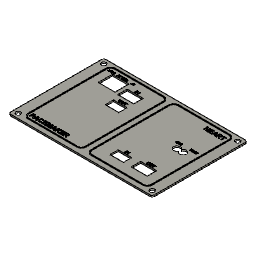
testing_station_casing_top v22 (Autodesk Fusion 360 design; units mm, degrees)
Autodesk Fusion 360 part; units mm, degrees
(part 1 of 2)
sketch "Sketch1" plane through (0, 0, 0) normal (0, 0, 1) x (1, 0, 0)
  line L0 (0, 0) -> (148, 0)
  line L1 (148, 0) -> (148, 98)
  line L2 (148, 98) -> (0, 98)
  line L3 (0, 98) -> (0, 0)
  dimension "d1" = 148
  dimension "d2" = 98
  constraint horizontal L0
  constraint vertical L1
  constraint horizontal L2
  constraint vertical L3
  constraint coincident L0.start L3.end
  measures "d1" distance of L0.start L0.end
  measures "d2" distance of L0.start L2.end
extrude "Extrude1" add sketch "Sketch1" along normal blind 1.5
sketch "Sketch2" plane through (0, 0, 1.5) normal (0, 0, 1) x (-1, 0, 0)
  line L0 (0, -98) -> (0, 0)
  line L1 (0, 0) -> (-148, 0)
  line L2 (-148, 0) -> (-148, -98)
  line L3 (-148, -98) -> (0, -98)
  line L4 (-7.1651, -89.25) -> (-2.8349, -89.25)
  line L5 (0, 0) -> (-148, 0)
  line L6 (-2.8349, -96.75) -> (-7.1651, -96.75)
  line L7 (0, -98) -> (0, 0)
  line L8 (-148, -98) -> (0, -98)
  line L9 (-2.8349, -89.25) -> (-0.6699, -93)
  line L10 (-9.3301, -93) -> (-7.1651, -89.25)
  line L11 (-148, 0) -> (-148, -98)
  line L12 (-0.6699, -93) -> (-2.8349, -96.75)
  line L13 (-7.1651, -96.75) -> (-9.3301, -93)
  circle A0 centre (-5, -93) radius 2.45
  circle A1 centre (-5, -5) radius 2.45
  circle A2 centre (-143, -5) radius 2.45
  circle A3 centre (-143, -93) radius 2.45
  dimension "d5" = 4.9
  dimension "d10" = 7.5
  dimension "d11" = 7.5
  dimension "d12" = 120
  dimension "d13" = 120
  dimension "d26" = 5
  dimension "d27" = 5
  dimension "d34" = 4.9
  dimension "d35" = 4.9
  dimension "d36" = 4.9
  dimension "d37" = 5
  dimension "d38" = 5
  dimension "d39" = 5
  dimension "d40" = 5
  dimension "d41" = 5
  dimension "d42" = 5
  dimension "d97" = 3.75
  dimension "d98" = 3.75
  dimension "d99" = 3.75
  constraint horizontal L6
  constraint parallel L4 L6
  constraint parallel L10 L12
  constraint parallel L9 L13
  constraint coincident L2.end L3.start
  constraint coincident L1.end L2.start
  constraint coincident L0.start L3.end
  constraint coincident L0.end L1.start
  constraint equal L9 L13
  measures "d5" diameter of A0
  measures "d10" distance of L10 L12
  measures "d11" distance of L9 L13
  measures "d12" angle of L4 L10
  measures "d13" angle of L6 L13
  measures "d26" distance of A0.centre L7
  measures "d27" distance of A0.centre L8
  measures "d34" diameter of A3
  measures "d35" diameter of A1
  measures "d36" diameter of A2
  measures "d37" distance of L11 A3.centre
  measures "d38" distance of L8 A3.centre
  measures "d39" distance of L11 A2.centre
  measures "d40" distance of L5 A2.centre
  measures "d41" distance of L5 A1.centre
  measures "d42" distance of L7 A1.centre
  measures "d97" distance of A0.centre L6
  measures "d98" distance of A0.centre L12
  measures "d99" distance of A0.centre L9
extrude "Extrude2" cut sketch "Sketch2" along normal through all and the other way through all contours A0 | A1 | A2 | A3
sketch "Sketch3" plane through (0, 0, 1.5) normal (0, 0, 1) x (-1, 0, 0)
  circle A0 centre (-5, -5) radius 2.45
  circle A1 centre (-5, -93) radius 2.45
  line L0 (0, -98) -> (0, 0)
  line L1 (-22.5, -92.78) -> (-22.5, -86.78)
  line L2 (-15, -86.78) -> (-15, -92.78)
  line L3 (-44.6822, -95.28) -> (-44.6822, -73.28)
  line L4 (-28.9322, -95.28) -> (-44.6822, -95.28)
  line L5 (-55.9389, -86.78) -> (-48.4389, -86.78)
  line L6 (-48.4389, -86.78) -> (-48.4389, -92.78)
  circle A2 centre (-12.8194, -22.6238) radius 1.5
  line L7 (-44.6822, -73.28) -> (-28.9322, -73.28)
  line L8 (-28.9322, -73.28) -> (-28.9322, -95.28)
  line L9 (-15, -92.78) -> (-22.5, -92.78)
  circle A3 centre (-59.7586, -77.5513) radius 1.5
  line L10 (-48.4389, -92.78) -> (-55.9389, -92.78)
  line L11 (-22.5, -86.78) -> (-15, -86.78)
  line L12 (-63.34, -10) -> (-10, -10)
  line L13 (-63.34, -91.28) -> (-63.34, -10)
  circle A4 centre (-12.8194, -76.3321) radius 1.5
  line L14 (-55.9389, -92.78) -> (-55.9389, -86.78)
  circle A5 centre (-59.7586, -22.6238) radius 1.5
  line L15 (-10, -91.28) -> (-63.34, -91.28)
  line L16 (-10, -10) -> (-10, -91.28)
  line L17 (0, 0) -> (-148, 0)
  line L18 (-148, 0) -> (-148, -98)
  line L19 (-148, -98) -> (0, -98)
  line L20 (0, -98) -> (0, 0)
  line L21 (-70.214, -90.398) -> (-140, -90.398)
  line L22 (-140, -90.398) -> (-140, -10)
  line L23 (-70.214, -10) -> (-70.214, -90.398)
  line L24 (-114.82, -91.7786) -> (-124.1322, -91.7786)
  line L25 (-124.1322, -91.7786) -> (-124.1322, -84.0185)
  line L26 (-124.1322, -84.0185) -> (-114.82, -84.0185)
  line L27 (-114.82, -84.0185) -> (-114.82, -91.7786)
  line L28 (-81.756, -10) -> (-83.5436, -8)
  line L29 (-83.5436, -8) -> (-116.4586, -8)
  line L30 (-116.4586, -8) -> (-118.458, -10)
  line L31 (-140, -10) -> (-118.458, -10)
  line L32 (-81.756, -10) -> (-70.214, -10)
  circle A6 centre (-113.89, -10.5) radius 1.5
  circle A7 centre (-129.13, -61.198) radius 1.5
  circle A8 centre (-81.084, -62.468) radius 1.5
  circle A9 centre (-129.13, -57.642) radius 1
  line L33 (-133.506, -56.3529) -> (-136.9699, -56.3529) construction
  line L34 (-136.9699, -56.3529) -> (-136.9699, -58.3529) construction
  line L35 (-136.9699, -58.3529) -> (-133.506, -58.3529) construction
  line L36 (-133.506, -58.3529) -> (-133.506, -56.3529) construction
  circle A10 centre (-60.6896, -73.1803) radius 1
  line L37 (-55.7149, -72.2742) -> (-59.1788, -72.2742) construction
  line L38 (-59.1788, -72.2742) -> (-59.1788, -74.2742) construction
  line L39 (-59.1788, -74.2742) -> (-55.7149, -74.2742) construction
  line L40 (-55.7149, -74.2742) -> (-55.7149, -72.2742) construction
  point P0 (-148, -98)
  dimension "d45" = 3
  dimension "d46" = 3
  dimension "d60" = 4
  dimension "d61" = 15.75
  dimension "d62" = 7.4011
  dimension "d63" = 53.34
  dimension "d64" = 81.28
  dimension "d65" = 18.6578
  dimension "d68" = 2.8194
  dimension "d69" = 14.9479
  dimension "d70" = 12.6238
  dimension "d73" = 2.8194
  dimension "d74" = 6
  dimension "d75" = 22
  dimension "d76" = 7.5
  dimension "d78" = 5
  dimension "d155" = 10
  dimension "d156" = 10
  dimension "d157" = 3
  dimension "d158" = 3
  dimension "d159" = 3.5814
  dimension "d160" = 54.9275
  dimension "d161" = 12.6238
  dimension "d162" = 3.5814
  dimension "d163" = 7.5
  dimension "d164" = 1.5
  dimension "d165" = 6
  dimension "d166" = 69.786
  dimension "d167" = 8
  dimension "d168" = 80.398
  dimension "d169" = 2
  dimension "d170" = 21.542
  dimension "d171" = 32.915
  dimension "d172" = 11.542
  dimension "d173" = 2.828
  dimension "d174" = 10.87
  dimension "d175" = 10.87
  dimension "d176" = 27.93
  dimension "d177" = 29.2
  dimension "d178" = 3
  dimension "d179" = 3
  dimension "d180" = 3
  dimension "d181" = 2.5
  dimension "d182" = 26.11
  dimension "d183" = 10
  dimension "d184" = 2
  dimension "d186" = 3.556
  dimension "d204" = 2
  dimension "d206" = 0.931
  dimension "d207" = 4.371
  constraint horizontal L15
  constraint vertical L13
  constraint horizontal L12
  constraint vertical L16
  constraint horizontal L10
  constraint vertical L14
  constraint horizontal L5
  constraint vertical L6
  constraint horizontal L4
  constraint vertical L3
  constraint horizontal L7
  constraint vertical L8
  constraint horizontal L9
  constraint horizontal L11
  constraint vertical L2
  constraint collinear L9 L10
  constraint collinear L5 L11
  constraint coincident L0.end L17.start
  constraint horizontal L17
  constraint vertical L18
  constraint horizontal L19
  constraint vertical L20
  constraint coincident P0 L18.end
  constraint horizontal L21
  constraint vertical L22
  constraint horizontal L31
  constraint vertical L23
  constraint horizontal L24
  constraint vertical L25
  constraint horizontal L26
  constraint vertical L27
  constraint coincident L28.start L31
  constraint collinear L31 L32
  constraint perpendicular L33 L34
  constraint parallel L33 L35
  constraint parallel L34 L36
  constraint vertical A7.centre A9.centre
  constraint perpendicular L37 L38
  constraint parallel L37 L39
  constraint parallel L38 L40
  measures "d45" diameter of A4
  measures "d46" diameter of A2
  measures "d60" distance of L4 L15
  measures "d61" distance of L4.start L3.start
  measures "d62" distance of L13 L14
  measures "d63" distance of L13.start L15.start
  measures "d64" distance of L15.start L12.end
  measures "d65" distance of L3 L13
  measures "d68" distance of A4.centre L16
  measures "d69" distance of A4.centre L15
  measures "d70" distance of A2.centre L12
  measures "d73" distance of A2.centre L16
  measures "d74" distance of L10.end L5.start
  measures "d75" distance of L7.end L4.start
  measures "d76" distance of L10.end L6.end
  measures "d78" distance of L2 L16
  measures "d155" distance of L16 L20
  measures "d156" distance of L12 L17
  measures "d157" diameter of A5
  measures "d158" diameter of A3
  measures "d159" distance of A3.centre L13
  measures "d160" distance of A3.centre A5.centre
  measures "d161" distance of A5.centre L12
  measures "d162" distance of A5.centre L13
  measures "d163" distance of L1.start L2.end
  measures "d164" distance of L9 L15
  measures "d165" distance of L1.end L1.start
  measures "d166" distance of L21.start L21.end
  measures "d167" distance of L18 L22
  measures "d168" distance of L21.end L22.end
  measures "d169" distance of L29 L31
  measures "d170" distance of L22 L30.end
  measures "d171" distance of L28.end L29.end
  measures "d172" distance of L23 L28.start
  measures "d173" distance of L29.end L30.end
  measures "d174" distance of L22 A7.centre
  measures "d175" distance of L23 A8.centre
  measures "d176" distance of L21 A8.centre
  measures "d177" distance of L21 A7.centre
  measures "d178" diameter of A8
  measures "d179" diameter of A7
  measures "d180" diameter of A6
  measures "d181" distance of L29 A6.centre
  measures "d182" distance of L22 A6.centre
  measures "d183" distance of L17 L31
  measures "d184" diameter of A9
  measures "d186" distance of A7.centre A9.centre
  measures "d204" diameter of A10
  measures "d206" horizontal distance of A3.centre A10.centre
  measures "d207" vertical distance of A3.centre A10.centre
sketch "Sketch4" plane through (0, 0, 1.5) normal (0, 0, 1) x (-1, 0, 0)
  line L0 (-41.7296, -80.5083) -> (-54.1296, -80.5083)
  line L1 (-54.1296, -80.5083) -> (-54.1296, -74.7583)
  line L2 (-54.1296, -74.7583) -> (-41.7296, -74.7583)
  line L3 (-41.7296, -74.7583) -> (-41.7296, -80.5083)
  line L4 (-44.2616, -63.8513) -> (-54.1616, -63.8513)
  line L5 (-54.1616, -63.8513) -> (-54.1616, -59.3513)
  line L6 (-54.1616, -59.3513) -> (-44.2616, -59.3513)
  line L7 (-44.2616, -59.3513) -> (-44.2616, -63.8513)
  line L8 (-113.193, -22.958) -> (-125.593, -22.958)
  line L9 (-125.593, -22.958) -> (-125.593, -17.208)
  line L10 (-125.593, -17.208) -> (-113.193, -17.208)
  line L11 (-113.193, -17.208) -> (-113.193, -22.958)
  line L12 (-91.149, -21.75) -> (-101.049, -21.75)
  line L13 (-101.049, -21.75) -> (-101.049, -17.25)
  line L14 (-101.049, -17.25) -> (-91.149, -17.25)
  line L15 (-91.149, -17.25) -> (-91.149, -21.75)
  line L16 (-103.049, -23.75) -> (-103.049, -15.25)
  line L17 (-103.049, -15.25) -> (-89.149, -15.25)
  line L18 (-89.149, -15.25) -> (-89.149, -23.75)
  line L19 (-89.149, -23.75) -> (-103.049, -23.75)
  line L20 (-111.193, -15.208) -> (-111.193, -24.958)
  line L21 (-111.193, -24.958) -> (-127.593, -24.958)
  line L22 (-127.593, -24.958) -> (-127.593, -15.208)
  line L23 (-127.593, -15.208) -> (-111.193, -15.208)
  line L24 (-39.7296, -72.7583) -> (-39.7296, -82.5083)
  line L25 (-39.7296, -82.5083) -> (-56.1296, -82.5083)
  line L26 (-56.1296, -82.5083) -> (-56.1296, -72.7583)
  line L27 (-56.1296, -72.7583) -> (-39.7296, -72.7583)
  line L28 (-42.2616, -65.8513) -> (-56.1616, -65.8513)
  line L29 (-56.1616, -65.8513) -> (-56.1616, -57.3513)
  line L30 (-56.1616, -57.3513) -> (-42.2616, -57.3513)
  line L31 (-42.2616, -57.3513) -> (-42.2616, -65.8513)
  line L32 (-20.8196, -75.5813) -> (-34.0196, -75.5813)
  line L33 (-34.0196, -75.5813) -> (-34.0196, -86.0963)
  line L34 (-34.0196, -86.0963) -> (-20.8196, -86.0963)
  line L35 (-20.8196, -86.0963) -> (-20.8196, -75.5813)
  line L36 (-36.0196, -88.0963) -> (-18.8196, -88.0963)
  line L37 (-18.8196, -88.0963) -> (-18.8196, -73.5813)
  line L38 (-18.8196, -73.5813) -> (-36.0196, -73.5813)
  line L39 (-36.0196, -73.5813) -> (-36.0196, -88.0963)
  circle A0 centre (-118.398, -55.077) radius 3.5
  circle A1 centre (-124.685, -55.077) radius 3.5
  point P0 (-129.13, -57.642)
  point P1 (-60.6896, -73.1803)
  dimension "d187" = 3.537
  dimension "d188" = 34.684
  dimension "d189" = 12.144
  dimension "d190" = 12.4
  dimension "d191" = 5.75
  dimension "d192" = 9.9
  dimension "d193" = 4.5
  dimension "d198" = -2
  dimension "d199" = -2
  dimension "d208" = 6.56
  dimension "d209" = 5.75
  dimension "d210" = 12.4
  dimension "d211" = 1.578
  dimension "d212" = 9.329
  dimension "d213" = 4.5
  dimension "d214" = 9.9
  dimension "d215" = 6.528
  dimension "d216" = -2
  dimension "d217" = -2
  dimension "d227" = 13.2
  dimension "d228" = 10.515
  dimension "d229" = 2
  dimension "d230" = 26.67
  dimension "d231" = 2.401
  dimension "d235" = 7
  dimension "d236" = 7
  dimension "d244" = 1.208
  dimension "d245" = 2.565
  dimension "d246" = 4.445
  dimension "d247" = 6.287
  constraint horizontal L0
  constraint vertical L1
  constraint horizontal L2
  constraint vertical L3
  constraint horizontal L4
  constraint vertical L5
  constraint horizontal L6
  constraint vertical L7
  constraint horizontal L8
  constraint vertical L9
  constraint horizontal L10
  constraint vertical L11
  constraint horizontal L12
  constraint vertical L13
  constraint horizontal L14
  constraint vertical L15
  constraint horizontal L32
  constraint vertical L33
  constraint horizontal L34
  constraint vertical L35
  constraint horizontal A0.centre A1.centre
  measures "d187" distance of L9 P0
  measures "d188" distance of L8 P0
  measures "d189" distance of L11 L13
  measures "d190" distance of L8.start L8.end
  measures "d191" distance of L8.start L10.end
  measures "d192" distance of L12.start L12.end
  measures "d193" distance of L12.start L14.end
  measures "d208" distance of L1 P1
  measures "d209" distance of L0.end L1.end
  measures "d210" distance of L0.start L0.end
  measures "d211" distance of L2 P1
  measures "d212" distance of L4 P1
  measures "d213" distance of L4.start L6.end
  measures "d214" distance of L5.end L6.end
  measures "d215" distance of L5 P1
  measures "d227" distance of L32.start L32.end
  measures "d228" distance of L32.start L34.end
  measures "d230" distance of P1 L33
  measures "d231" distance of P1 L32
  measures "d235" diameter of A1
  measures "d236" diameter of A0
  measures "d244" distance of L8 L12
  measures "d245" vertical distance of P0 A1.centre
  measures "d246" horizontal distance of P0 A1.centre
  measures "d247" distance of A0.centre A1.centre
extrude "Extrude3" cut sketch "Sketch4" along normal through all and the other way through all contours L0 L1 L2 L3 | L4 L5 L6 L7 | L8 L9 L10 L11 | L12 L13 L14 L15 | L16 L17 L18 L19 | L20 L21 L22 L23 | L24 L25 L26 L27 | L28 L29 L30 L31 | L32 L33 L34 L35 | L36 L37 L38 L39 | A0 A1 | A0 A1 | A0 A1
sketch "Sketch5" plane through (0, 0, 1.5) normal (0, 0, 1) x (-1, 0, 0)
  circle A0 centre (-5, -5) radius 2.45
  circle A1 centre (-143, -5) radius 2.45
  circle A2 centre (-5, -93) radius 2.45
  circle A3 centre (-143, -93) radius 2.45
  line L0 (0, -98) -> (0, 0)
  line L1 (0, 0) -> (-148, 0)
  line L2 (-148, 0) -> (-148, -98)
  line L3 (-148, -98) -> (0, -98)
  line L4 (-46.2265, -83.5083) -> (-49.6327, -83.5083) construction
  line L5 (-49.6327, -83.5083) -> (-49.6327, -87.5083) construction
  line L6 (-49.6327, -87.5083) -> (-46.2265, -87.5083) construction
  line L7 (-46.2265, -87.5083) -> (-46.2265, -83.5083) construction
  line L8 (-45.1178, -66.8513) -> (-53.3053, -66.8513) construction
  line L9 (-53.3053, -66.8513) -> (-53.3053, -70.8513) construction
  line L10 (-53.3053, -70.8513) -> (-45.1178, -70.8513) construction
  line L11 (-45.1178, -70.8513) -> (-45.1178, -66.8513) construction
  line L12 (-115.2993, -25.958) -> (-123.4868, -25.958) construction
  line L13 (-123.4868, -25.958) -> (-123.4868, -29.958) construction
  line L14 (-123.4868, -29.958) -> (-115.2993, -29.958) construction
  line L15 (-115.2993, -29.958) -> (-115.2993, -25.958) construction
  line L16 (-94.3959, -24.75) -> (-97.8021, -24.75) construction
  line L17 (-97.8021, -24.75) -> (-97.8021, -28.75) construction
  line L18 (-97.8021, -28.75) -> (-94.3959, -28.75) construction
  line L19 (-94.3959, -28.75) -> (-94.3959, -24.75) construction
  line L20 (-22.1066, -89.0963) -> (-32.7326, -89.0963) construction
  line L21 (-32.7326, -89.0963) -> (-32.7326, -92.0963) construction
  line L22 (-32.7326, -92.0963) -> (-22.1066, -92.0963) construction
  line L23 (-22.1066, -92.0963) -> (-22.1066, -89.0963) construction
  line L24 (-13.0194, -89.0963) -> (-19.5277, -89.0963) construction
  line L25 (-19.5277, -89.0963) -> (-19.5277, -92.0963) construction
  line L26 (-19.5277, -92.0963) -> (-13.0194, -92.0963) construction
  line L27 (-13.0194, -92.0963) -> (-13.0194, -89.0963) construction
  line L28 (-36.486, -89.0963) -> (-39.8325, -89.0963) construction
  line L29 (-39.8325, -89.0963) -> (-39.8325, -92.0963) construction
  line L30 (-39.8325, -92.0963) -> (-36.486, -92.0963) construction
  line L31 (-36.486, -92.0963) -> (-36.486, -89.0963) construction
  line L32 (-27.4196, -88.0963) -> (-27.4196, -73.5813)
  line L33 (-127.593, -15.208) -> (-111.193, -15.208)
  line L34 (-111.193, -15.208) -> (-111.193, -24.958)
  line L35 (-111.193, -24.958) -> (-127.593, -24.958)
  line L36 (-127.593, -24.958) -> (-127.593, -15.208)
  line L37 (-89.149, -23.75) -> (-103.049, -23.75)
  line L38 (-103.049, -23.75) -> (-103.049, -15.25)
  line L39 (-103.049, -15.25) -> (-89.149, -15.25)
  line L40 (-89.149, -15.25) -> (-89.149, -23.75)
  line L41 (-89.149, -15.25) -> (-89.149, -23.75)
  line L42 (-42.2616, -57.3513) -> (-42.2616, -65.8513)
  line L43 (-42.2616, -65.8513) -> (-56.1616, -65.8513)
  line L44 (-56.1616, -65.8513) -> (-56.1616, -57.3513)
  line L45 (-56.1616, -57.3513) -> (-42.2616, -57.3513)
  line L46 (-56.1296, -72.7583) -> (-39.7296, -72.7583)
  line L47 (-39.7296, -72.7583) -> (-39.7296, -82.5083)
  line L48 (-39.7296, -82.5083) -> (-56.1296, -82.5083)
  line L49 (-56.1296, -82.5083) -> (-56.1296, -72.7583)
  line L50 (-39.7296, -72.7583) -> (-39.7296, -82.5083)
  line L51 (-42.2616, -57.3513) -> (-42.2616, -65.8513)
  line L52 (-36.0196, -73.5813) -> (-18.8196, -73.5813)
  line L53 (-18.8196, -73.5813) -> (-18.8196, -88.0963)
  line L54 (-18.8196, -88.0963) -> (-36.0196, -88.0963)
  line L55 (-36.0196, -88.0963) -> (-36.0196, -73.5813)
  line L56 (-111.398, -60.077) -> (-117.398, -60.077) construction
  line L57 (-117.398, -60.077) -> (-117.398, -63.077) construction
  line L58 (-117.398, -63.077) -> (-111.398, -63.077) construction
  line L59 (-111.398, -63.077) -> (-111.398, -60.077) construction
  line L60 (-125.685, -60.077) -> (-135.72, -60.077) construction
  line L61 (-135.72, -60.077) -> (-135.72, -63.077) construction
  line L62 (-135.72, -63.077) -> (-125.685, -63.077) construction
  line L63 (-125.685, -63.077) -> (-125.685, -60.077) construction
  arc A4 (-121.5415, -56.616) -> (-121.5415, -53.538) centre (-118.398, -55.077) ccw
  arc A5 (-121.5415, -53.538) -> (-121.5415, -56.616) centre (-124.685, -55.077) ccw
  dimension "d124" = 3.4062
  dimension "d126" = 8.1875
  dimension "d127" = 4
  dimension "d128" = 4
  dimension "d132" = 8.1875
  dimension "d133" = 4
  dimension "d134" = 4
  dimension "d135" = 3.4062
  dimension "d147" = 3
  dimension "d149" = 3.3465
  dimension "d151" = 6.5083
  dimension "d153" = 10.626
  dimension "d154" = 5.313
  dimension "d200" = 1
  dimension "d201" = 1
  dimension "d202" = 4.1063
  dimension "d203" = 5.2469
  dimension "d218" = 1
  dimension "d219" = 1
  dimension "d220" = 6.4969
  dimension "d221" = 2.8563
  dimension "d232" = 1
  dimension "d237" = 3
  dimension "d239" = 1
  dimension "d240" = 5
  dimension "d242" = 6
  dimension "d248" = 1
  dimension "d249" = 5
  text T0 "IN" font "Arial" height 4 bold align ink ink in box 0 x 0 at (-46.2265, -83.5083) x (-1, 0) y (0, -1) spacing 1 height is em
  text T1 "OUT" font "Arial" height 4 bold align ink ink in box 0 x 0 at (-45.1178, -66.8513) x (-1, 0) y (0, -1) spacing 1 height is em
  text T2 "OUT" font "Arial" height 4 bold align ink ink in box 0 x 0 at (-115.2993, -25.958) x (-1, 0) y (0, -1) spacing 1 height is em
  text T3 "IN" font "Arial" height 4 bold align ink ink in box 0 x 0 at (-94.3959, -24.75) x (-1, 0) y (0, -1) spacing 1 height is em
  text T4 "ATTEN." font "Arial" height 3 bold align ink ink in box 0 x 0 at (-22.1066, -89.0963) x (-1, 0) y (0, -1) spacing 1 height is em
  text T5 "x100" font "Arial" height 3 bold align ink ink in box 0 x 0 at (-13.0194, -89.0963) x (-1, 0) y (0, -1) spacing 1 height is em
  text T6 "x1" font "Arial" height 3 bold align ink ink in box 0 x 0 at (-36.486, -89.0963) x (-1, 0) y (0, -1) spacing 1 height is em
  text T7 "ATR" font "Arial" height 3 bold align ink ink in box 0 x 0 at (-111.398, -60.077) x (-1, 0) y (0, -1) spacing 1 height is em
  text T8 "VENT" font "Arial" height 3 bold align ink ink in box 0 x 0 at (-125.685, -60.077) x (-1, 0) y (0, -1) spacing 1 height is em
  constraint perpendicular L4 L5
  constraint parallel L4 L6
  constraint parallel L5 L7
  constraint perpendicular L8 L9
  constraint parallel L8 L10
  constraint parallel L9 L11
  constraint perpendicular L12 L13
  constraint parallel L12 L14
  constraint parallel L13 L15
  constraint perpendicular L16 L17
  constraint parallel L16 L18
  constraint parallel L17 L19
  constraint perpendicular L20 L21
  constraint parallel L20 L22
  constraint parallel L21 L23
  constraint perpendicular L24 L25
  constraint parallel L24 L26
  constraint parallel L25 L27
  constraint perpendicular L28 L29
  constraint parallel L28 L30
  constraint parallel L29 L31
  constraint collinear L22 L26
  constraint collinear L22 L30
  constraint collinear L20 L24
  constraint collinear L20 L28
  constraint coincident L32.start L54
  constraint coincident L32.end L52
  constraint perpendicular L32 L52
  constraint midpoint L32.end L52
  constraint perpendicular L56 L57
  constraint parallel L56 L58
  constraint parallel L57 L59
  constraint perpendicular L60 L61
  constraint parallel L60 L62
  constraint parallel L61 L63
  constraint collinear L58 L62
  constraint collinear L56 L60
  constraint parallel L3 L56
  measures "d124" distance of L5.end L6.end
  measures "d126" distance of L9.end L10.end
  measures "d127" distance of L4.end L5.end
  measures "d128" distance of L8.end L9.end
  measures "d132" distance of L13.end L14.end
  measures "d133" distance of L12.end L13.end
  measures "d134" distance of L16.end L17.end
  measures "d135" distance of L17.end L18.end
  measures "d147" distance of L24.start L26.end
  measures "d149" distance of L29.end L30.end
  measures "d151" distance of L25.end L26.end
  measures "d153" distance of L21.end L22.end
  measures "d154" distance of L23 L32
  measures "d200" distance of L16 L37
  measures "d201" distance of L12 L35
  measures "d202" distance of L15 L34
  measures "d203" distance of L19 L41
  measures "d218" distance of L8 L43
  measures "d219" distance of L4 L48
  measures "d220" distance of L7 L50
  measures "d221" distance of L11 L51
  measures "d232" distance of L20 L54
  measures "d237" distance of L56.start L58.end
  measures "d239" distance of L57 A4.centre
  measures "d242" distance of L57.end L58.end
  measures "d248" distance of L63 A5.centre
  measures "d249" distance of L56 A4.centre
extrude "Extrude4" cut sketch "Sketch5" against normal blind 0.5 text T0 T1 T2 T3 T5 T4 T6 T7 T8
fillet "Fillet1" radius 2 4 edges at (0, 0, 0.75) (148, 0, 0.75) (148, 98, 0.75) (0, 98, 0.75)
sketch "Sketch6" plane through (0, 0, 1.5) normal (0, 0, 1) x (-1, 0, 0)
  spline S0 degree 3 poles (-120.2604, -26.0639) (-120.18, -26.0389) (-120.0008, -25.9833) (-119.8131, -25.9799) (-119.7096, -25.978) knots 0 0 0 0 0.025156 0.055993 0.055993 0.055993 0.055993
  spline S1 degree 3 poles (-119.7096, -25.978) (-119.5883, -25.9791) (-119.3757, -25.9811) (-119.1734, -26.0445) (-119.0866, -26.0718) knots 0 0 0 0 0.03616 0.063307 0.063307 0.063307 0.063307
  spline S2 degree 3 poles (-119.0866, -26.0718) (-119.021, -26.1047) (-118.8955, -26.1677) (-118.7988, -26.2693) (-118.7526, -26.3178) knots 0 0 0 0 0.021834 0.041764 0.041764 0.041764 0.041764
  spline S3 degree 3 poles (-118.7526, -26.3178) (-118.7154, -26.3681) (-118.6434, -26.4652) (-118.6077, -26.5806) (-118.5905, -26.6362) knots 0 0 0 0 0.018622 0.035955 0.035955 0.035955 0.035955
  spline S4 degree 3 poles (-118.5905, -26.6362) (-118.5741, -26.7376) (-118.5351, -26.978) (-118.5343, -27.2218) (-118.5339, -27.3628) knots 0 0 0 0 0.030763 0.072975 0.072975 0.072975 0.072975
  line L0 (-118.5339, -27.3628) -> (-118.5339, -28.8901)
  line L1 (-121.2214, -28.4057) -> (-121.2214, -28.8901)
  spline S5 degree 3 poles (-49.1279, -67.4709) (-49.1819, -67.4402) (-49.3002, -67.373) (-49.4366, -67.3681) (-49.5107, -67.3654) knots 0 0 0 0 0.01839 0.040229 0.040229 0.040229 0.040229
  spline S6 degree 3 poles (-49.5107, -67.3654) (-49.5845, -67.3673) (-49.7168, -67.3706) (-49.8312, -67.4361) (-49.8818, -67.465) knots 0 0 0 0 0.021725 0.038956 0.038956 0.038956 0.038956
  spline S7 degree 3 poles (-49.8818, -67.465) (-49.9192, -67.5002) (-49.9924, -67.569) (-50.0191, -67.6658) (-50.0321, -67.7131) knots 0 0 0 0 0.01508 0.029511 0.029511 0.029511 0.029511
  spline S8 degree 3 poles (-50.0321, -67.7131) (-50.0395, -67.778) (-50.0578, -67.9395) (-50.0576, -68.1021) (-50.0575, -68.1994) knots 0 0 0 0 0.019575 0.048733 0.048733 0.048733 0.048733
  line L2 (-50.0575, -69.7834) -> (-50.6357, -69.7834)
  spline S9 degree 3 poles (-50.6357, -68.2795) (-50.6359, -68.1325) (-50.6364, -67.8885) (-50.6023, -67.647) (-50.5888, -67.551) knots 0 0 0 0 0.04401 0.073081 0.073081 0.073081 0.073081
  spline S10 degree 3 poles (-50.415, -67.1916) (-50.3683, -67.1446) (-50.2705, -67.0463) (-50.1447, -66.9878) (-50.079, -66.9572) knots 0 0 0 0 0.019707 0.04125 0.04125 0.04125 0.04125
  spline S11 degree 3 poles (-50.079, -66.9572) (-49.9986, -66.9322) (-49.8194, -66.8766) (-49.6317, -66.8732) (-49.5282, -66.8713) knots 0 0 0 0 0.025156 0.055993 0.055993 0.055993 0.055993
  spline S12 degree 3 poles (-49.5282, -66.8713) (-49.4069, -66.8724) (-49.1943, -66.8744) (-48.992, -66.9378) (-48.9052, -66.9651) knots 0 0 0 0 0.03616 0.063307 0.063307 0.063307 0.063307
  spline S13 degree 3 poles (-48.9052, -66.9651) (-48.8396, -66.998) (-48.7141, -67.061) (-48.6174, -67.1626) (-48.5712, -67.2111) knots 0 0 0 0 0.021834 0.041764 0.041764 0.041764 0.041764
  spline S14 degree 3 poles (-48.5712, -67.2111) (-48.534, -67.2614) (-48.462, -67.3585) (-48.4263, -67.4739) (-48.4091, -67.5295) knots 0 0 0 0 0.018622 0.035955 0.035955 0.035955 0.035955
  spline S15 degree 3 poles (-48.4091, -67.5295) (-48.3927, -67.6309) (-48.3537, -67.8713) (-48.3529, -68.1151) (-48.3525, -68.2561) knots 0 0 0 0 0.030763 0.072975 0.072975 0.072975 0.072975
  line L3 (-51.04, -69.7834) -> (-53.3154, -69.7834)
  line L4 (-47.9084, -85.3955) -> (-47.9084, -83.5283)
  line L5 (-49.6427, -83.5283) -> (-49.0626, -83.5283)
  line L6 (-49.0626, -83.5283) -> (-47.9084, -85.3955)
  line L7 (-46.2365, -83.5283) -> (-46.2365, -86.3916)
  line L8 (-46.2365, -86.3916) -> (-46.8146, -86.3916)
  line L9 (-46.8146, -86.3916) -> (-46.8146, -83.5283)
  line L10 (-46.8146, -83.5283) -> (-46.2365, -83.5283)
  line L11 (-47.3712, -83.5283) -> (-47.3712, -86.3916)
  line L12 (-47.3712, -86.3916) -> (-47.9337, -86.3916)
  line L13 (-47.9337, -86.3916) -> (-49.1056, -84.4795)
  line L14 (-49.1056, -84.4795) -> (-49.1056, -86.3916)
  line L15 (-49.1056, -86.3916) -> (-49.6427, -86.3916)
  line L16 (-49.6427, -86.3916) -> (-49.6427, -83.5283)
  spline S16 degree 3 poles (-45.5243, -69.4611) (-45.5813, -69.5149) (-45.6921, -69.6195) (-45.8289, -69.6864) (-45.8954, -69.719) knots 0 0 0 0 0.023346 0.045418 0.045418 0.045418 0.045418
  spline S17 degree 3 poles (-45.8954, -69.719) (-45.9906, -69.752) (-46.1903, -69.8213) (-46.4018, -69.8285) (-46.5126, -69.8322) knots 0 0 0 0 0.030035 0.063067 0.063067 0.063067 0.063067
  spline S18 degree 3 poles (-46.5126, -69.8322) (-46.7101, -69.8188) (-47.0891, -69.793) (-47.3834, -69.5541) (-47.5243, -69.4397) knots 0 0 0 0 0.057773 0.110914 0.110914 0.110914 0.110914
  spline S19 degree 3 poles (-47.5243, -69.4397) (-47.6353, -69.289) (-47.8734, -68.9655) (-47.8941, -68.5629) (-47.9052, -68.3479) knots 0 0 0 0 0.054934 0.117914 0.117914 0.117914 0.117914
  spline S20 degree 3 poles (-47.9052, -68.3479) (-47.8942, -68.1344) (-47.8735, -67.7344) (-47.6381, -67.4122) (-47.5282, -67.2619) knots 0 0 0 0 0.062531 0.117188 0.117188 0.117188 0.117188
  spline S21 degree 3 poles (-47.5282, -67.2619) (-47.3879, -67.148) (-47.0948, -66.9102) (-46.7172, -66.8846) (-46.5204, -66.8713) knots 0 0 0 0 0.052897 0.11047 0.11047 0.11047 0.11047
  spline S22 degree 3 poles (-46.5204, -66.8713) (-46.3217, -66.8843) (-45.9419, -66.909) (-45.6459, -67.1467) (-45.5048, -67.26) knots 0 0 0 0 0.058142 0.111121 0.111121 0.111121 0.111121
  spline S23 degree 3 poles (-120.0632, -26.5717) (-120.1006, -26.6069) (-120.1738, -26.6757) (-120.2005, -26.7725) (-120.2135, -26.8198) knots 0 0 0 0 0.01508 0.029511 0.029511 0.029511 0.029511
  spline S24 degree 3 poles (-120.2135, -26.8198) (-120.2209, -26.8847) (-120.2392, -27.0462) (-120.239, -27.2088) (-120.2389, -27.3061) knots 0 0 0 0 0.019575 0.048733 0.048733 0.048733 0.048733
  spline S25 degree 3 poles (-119.112, -27.3393) (-119.1114, -27.2378) (-119.1104, -27.0778) (-119.1273, -26.9189) (-119.1335, -26.8608) knots 0 0 0 0 0.030425 0.047931 0.047931 0.047931 0.047931
  spline S26 degree 3 poles (-119.3093, -26.5776) (-119.3633, -26.5469) (-119.4816, -26.4797) (-119.618, -26.4748) (-119.6921, -26.4721) knots 0 0 0 0 0.01839 0.040229 0.040229 0.040229 0.040229
  spline S27 degree 3 poles (-119.6921, -26.4721) (-119.7659, -26.474) (-119.8982, -26.4773) (-120.0126, -26.5428) (-120.0632, -26.5717) knots 0 0 0 0 0.021725 0.038956 0.038956 0.038956 0.038956
  line L17 (-97.8121, -24.77) -> (-97.232, -24.77)
  line L18 (-97.232, -24.77) -> (-96.0778, -26.6372)
  line L19 (-94.4059, -24.77) -> (-94.4059, -27.6333)
  line L20 (-94.4059, -27.6333) -> (-94.984, -27.6333)
  line L21 (-97.8121, -27.6333) -> (-97.8121, -24.77)
  circle A0 centre (-5, -5) radius 2.45
  circle A1 centre (-143, -5) radius 2.45
  circle A2 centre (-5, -93) radius 2.45
  circle A3 centre (-143, -93) radius 2.45
  arc A4 (-2, -98) -> (0, -96) centre (-2, -96) ccw
  line L22 (0, -96) -> (0, -2)
  arc A5 (0, -2) -> (-2, 0) centre (-2, -2) ccw
  line L23 (-2, 0) -> (-146, 0)
  arc A6 (-146, 0) -> (-148, -2) centre (-146, -2) ccw
  line L24 (-148, -2) -> (-148, -96)
  arc A7 (-148, -96) -> (-146, -98) centre (-146, -96) ccw
  line L25 (-146, -98) -> (-2, -98)
  line L26 (-15, -95) -> (-65, -95)
  line L27 (-70, -90) -> (-70, -10)
  line L28 (-65, -5) -> (-15, -5)
  line L29 (-10, -10) -> (-10, -90)
  line L30 (-80, -95) -> (-133, -95)
  line L31 (-138, -90) -> (-138, -10)
  line L32 (-133, -5) -> (-80, -5)
  line L33 (-75, -10) -> (-75, -90)
  arc A8 (-15, -95) -> (-10, -90) centre (-15, -90) ccw
  arc A9 (-70, -90) -> (-65, -95) centre (-65, -90) ccw
  arc A10 (-80, -95) -> (-75, -90) centre (-80, -90) ccw
  arc A11 (-138, -90) -> (-133, -95) centre (-133, -90) ccw
  arc A12 (-133, -5) -> (-138, -10) centre (-133, -10) ccw
  arc A13 (-75, -10) -> (-80, -5) centre (-80, -10) ccw
  arc A14 (-65, -5) -> (-70, -10) centre (-65, -10) ccw
  arc A15 (-10, -10) -> (-15, -5) centre (-15, -10) ccw
  arc A16 (-15, -94) -> (-11, -90) centre (-15, -90) ccw
  line L34 (-11, -10) -> (-11, -90)
  arc A17 (-11, -10) -> (-15, -6) centre (-15, -10) ccw
  line L35 (-65, -6) -> (-15, -6)
  arc A18 (-65, -6) -> (-69, -10) centre (-65, -10) ccw
  line L36 (-69, -90) -> (-69, -10)
  arc A19 (-69, -90) -> (-65, -94) centre (-65, -90) ccw
  line L37 (-15, -94) -> (-65, -94)
  arc A20 (-80, -94) -> (-76, -90) centre (-80, -90) ccw
  line L38 (-76, -10) -> (-76, -90)
  arc A21 (-76, -10) -> (-80, -6) centre (-80, -10) ccw
  line L39 (-133, -6) -> (-80, -6)
  arc A22 (-133, -6) -> (-137, -10) centre (-133, -10) ccw
  line L40 (-137, -90) -> (-137, -10)
  arc A23 (-137, -90) -> (-133, -94) centre (-133, -90) ccw
  line L41 (-80, -94) -> (-133, -94)
  line L42 (-96.0778, -26.6372) -> (-96.0778, -24.77)
  line L43 (-96.0778, -24.77) -> (-95.5406, -24.77)
  line L44 (-95.5406, -24.77) -> (-95.5406, -27.6333)
  line L45 (-95.5406, -27.6333) -> (-96.1031, -27.6333)
  line L46 (-96.1031, -27.6333) -> (-97.275, -25.7212)
  line L47 (-97.275, -25.7212) -> (-97.275, -27.6333)
  line L48 (-97.275, -27.6333) -> (-97.8121, -27.6333)
  line L49 (-122.6491, -28.4057) -> (-122.6491, -26.0268)
  line L50 (-122.6491, -26.0268) -> (-122.071, -26.0268)
  line L51 (-122.071, -26.0268) -> (-122.071, -28.4057)
  line L52 (-122.071, -28.4057) -> (-121.2214, -28.4057)
  line L53 (-121.2214, -28.8901) -> (-123.4968, -28.8901)
  line L54 (-123.4968, -28.8901) -> (-123.4968, -28.4057)
  line L55 (-123.4968, -28.4057) -> (-122.6491, -28.4057)
  spline S28 degree 3 poles (-45.5048, -67.26) (-45.395, -67.4089) (-45.1603, -67.7271) (-45.1391, -68.1234) (-45.1279, -68.3342) knots 0 0 0 0 0.054323 0.116082 0.116082 0.116082 0.116082
  spline S29 degree 3 poles (-45.1279, -68.3342) (-45.1314, -68.4697) (-45.1381, -68.7214) (-45.2206, -68.9589) (-45.2587, -69.0686) knots 0 0 0 0 0.040367 0.07499 0.07499 0.07499 0.07499
  spline S30 degree 3 poles (-45.2587, -69.0686) (-45.2943, -69.1397) (-45.3655, -69.2822) (-45.4713, -69.4014) (-45.5243, -69.4611) knots 0 0 0 0 0.023737 0.047583 0.047583 0.047583 0.047583
  line L56 (-48.3525, -68.2561) -> (-48.3525, -69.7834)
  line L57 (-48.3525, -69.7834) -> (-48.9306, -69.7834)
  line L58 (-48.9306, -69.7834) -> (-48.9306, -68.2326)
  spline S31 degree 3 poles (-48.9306, -68.2326) (-48.93, -68.1311) (-48.929, -67.9711) (-48.9459, -67.8122) (-48.9521, -67.7541) knots 0 0 0 0 0.030425 0.047931 0.047931 0.047931 0.047931
  spline S32 degree 3 poles (-48.9521, -67.7541) (-48.9685, -67.6985) (-49.0012, -67.588) (-49.0858, -67.5098) (-49.1279, -67.4709) knots 0 0 0 0 0.017056 0.033889 0.033889 0.033889 0.033889
  line L59 (-50.0575, -68.1994) -> (-50.0575, -69.7834)
  line L60 (-50.6357, -69.7834) -> (-50.6357, -68.2795)
  spline S33 degree 3 poles (-50.5888, -67.551) (-50.5705, -67.4836) (-50.535, -67.3528) (-50.4542, -67.2442) (-50.415, -67.1916) knots 0 0 0 0 0.020737 0.040239 0.040239 0.040239 0.040239
  line L61 (-47.9084, -83.5283) -> (-47.3712, -83.5283)
  line L62 (-52.4677, -69.299) -> (-52.4677, -66.9201)
  line L63 (-52.4677, -66.9201) -> (-51.8896, -66.9201)
  line L64 (-51.8896, -66.9201) -> (-51.8896, -69.299)
  line L65 (-51.8896, -69.299) -> (-51.04, -69.299)
  line L66 (-51.04, -69.299) -> (-51.04, -69.7834)
  line L67 (-53.3154, -69.7834) -> (-53.3154, -69.299)
  line L68 (-53.3154, -69.299) -> (-52.4677, -69.299)
  line L69 (-118.5339, -28.8901) -> (-119.112, -28.8901)
  line L70 (-119.112, -28.8901) -> (-119.112, -27.3393)
  spline S34 degree 3 poles (-119.1335, -26.8608) (-119.1499, -26.8052) (-119.1826, -26.6947) (-119.2672, -26.6165) (-119.3093, -26.5776) knots 0 0 0 0 0.017056 0.033889 0.033889 0.033889 0.033889
  line L71 (-120.2389, -27.3061) -> (-120.2389, -28.8901)
  line L72 (-120.2389, -28.8901) -> (-120.8171, -28.8901)
  line L73 (-120.8171, -28.8901) -> (-120.8171, -27.3862)
  spline S35 degree 3 poles (-120.8171, -27.3862) (-120.8173, -27.2392) (-120.8178, -26.9952) (-120.7837, -26.7537) (-120.7702, -26.6577) knots 0 0 0 0 0.04401 0.073081 0.073081 0.073081 0.073081
  spline S36 degree 3 poles (-120.7702, -26.6577) (-120.7519, -26.5903) (-120.7164, -26.4595) (-120.6356, -26.3509) (-120.5964, -26.2983) knots 0 0 0 0 0.020737 0.040239 0.040239 0.040239 0.040239
  spline S37 degree 3 poles (-120.5964, -26.2983) (-120.5497, -26.2513) (-120.4519, -26.153) (-120.3261, -26.0945) (-120.2604, -26.0639) knots 0 0 0 0 0.019707 0.04125 0.04125 0.04125 0.04125
  spline S38 degree 3 poles (-116.7018, -25.978) (-116.5031, -25.991) (-116.1233, -26.0157) (-115.8273, -26.2534) (-115.6862, -26.3667) knots 0 0 0 0 0.058142 0.111121 0.111121 0.111121 0.111121
  spline S39 degree 3 poles (-115.6862, -26.3667) (-115.5764, -26.5156) (-115.3417, -26.8338) (-115.3205, -27.2301) (-115.3092, -27.4409) knots 0 0 0 0 0.054323 0.116082 0.116082 0.116082 0.116082
  spline S40 degree 3 poles (-115.3092, -27.4409) (-115.3128, -27.5764) (-115.3195, -27.8281) (-115.402, -28.0656) (-115.4401, -28.1753) knots 0 0 0 0 0.040367 0.07499 0.07499 0.07499 0.07499
  spline S41 degree 3 poles (-115.4401, -28.1753) (-115.4757, -28.2464) (-115.5469, -28.3889) (-115.6527, -28.5081) (-115.7057, -28.5678) knots 0 0 0 0 0.023737 0.047583 0.047583 0.047583 0.047583
  spline S42 degree 3 poles (-115.7057, -28.5678) (-115.7627, -28.6216) (-115.8735, -28.7262) (-116.0103, -28.7931) (-116.0768, -28.8257) knots 0 0 0 0 0.023346 0.045418 0.045418 0.045418 0.045418
  spline S43 degree 3 poles (-116.0768, -28.8257) (-116.172, -28.8587) (-116.3717, -28.928) (-116.5832, -28.9352) (-116.694, -28.9389) knots 0 0 0 0 0.030035 0.063067 0.063067 0.063067 0.063067
  spline S44 degree 3 poles (-116.694, -28.9389) (-116.8915, -28.9255) (-117.2705, -28.8997) (-117.5648, -28.6608) (-117.7057, -28.5464) knots 0 0 0 0 0.057773 0.110914 0.110914 0.110914 0.110914
  spline S45 degree 3 poles (-117.7057, -28.5464) (-117.8167, -28.3957) (-118.0548, -28.0722) (-118.0755, -27.6696) (-118.0866, -27.4546) knots 0 0 0 0 0.054934 0.117914 0.117914 0.117914 0.117914
  spline S46 degree 3 poles (-118.0866, -27.4546) (-118.0756, -27.2411) (-118.0549, -26.8411) (-117.8195, -26.5189) (-117.7096, -26.3686) knots 0 0 0 0 0.062531 0.117188 0.117188 0.117188 0.117188
  spline S47 degree 3 poles (-117.7096, -26.3686) (-117.5693, -26.2547) (-117.2762, -26.0169) (-116.8986, -25.9913) (-116.7018, -25.978) knots 0 0 0 0 0.052897 0.11047 0.11047 0.11047 0.11047
  line L74 (-94.984, -27.6333) -> (-94.984, -24.77)
  line L75 (-94.984, -24.77) -> (-94.4059, -24.77)
  line L76 (-37.2972, -89.5982) -> (-36.9779, -89.1163)
  line L77 (-36.9779, -89.1163) -> (-36.496, -89.1163)
  line L78 (-36.496, -89.1163) -> (-37.057, -89.9176)
  line L79 (-37.057, -89.9176) -> (-36.5194, -90.672)
  line L80 (-36.5194, -90.672) -> (-37.0218, -90.672)
  line L81 (-37.0218, -90.672) -> (-37.2972, -90.2442)
  line L82 (-37.2972, -90.2442) -> (-37.5873, -90.672)
  line L83 (-37.5873, -90.672) -> (-38.0707, -90.672)
  line L84 (-38.0707, -90.672) -> (-37.5433, -89.9351)
  line L85 (-37.5433, -89.9351) -> (-38.119, -89.1163)
  line L86 (-38.119, -89.1163) -> (-37.6136, -89.1163)
  line L87 (-37.6136, -89.1163) -> (-37.2972, -89.5982)
  line L88 (-22.953, -91.2638) -> (-23.4115, -91.2638)
  line L89 (-23.4115, -91.2638) -> (-24.2714, -89.1163)
  line L90 (-22.1166, -89.1163) -> (-22.953, -91.2638)
  line L91 (-27.2509, -90.9005) -> (-27.2509, -89.1163)
  line L92 (-26.8173, -89.1163) -> (-26.8173, -90.9005)
  line L93 (-26.8173, -90.9005) -> (-26.1801, -90.9005)
  line L94 (-26.1801, -90.9005) -> (-26.1801, -91.2638)
  line L95 (-26.1801, -91.2638) -> (-27.8866, -91.2638)
  line L96 (-27.8866, -91.2638) -> (-27.8866, -90.9005)
  line L97 (-27.8866, -90.9005) -> (-27.2509, -90.9005)
  line L98 (-28.1664, -89.1163) -> (-28.1664, -91.2638)
  line L99 (-28.1664, -91.2638) -> (-29.7587, -91.2638)
  line L100 (-29.7587, -91.2638) -> (-29.7587, -90.9005)
  line L101 (-29.7587, -90.9005) -> (-28.6, -90.9005)
  line L102 (-28.6, -90.9005) -> (-28.6, -90.4244)
  line L103 (-28.6, -90.4244) -> (-29.6781, -90.4244)
  line L104 (-29.6781, -90.4244) -> (-29.6781, -90.0626)
  line L105 (-29.6781, -90.0626) -> (-28.6, -90.0626)
  line L106 (-28.6, -90.0626) -> (-28.6, -89.4781)
  line L107 (-13.8306, -89.6349) -> (-13.5113, -89.1529)
  line L108 (-13.5113, -89.1529) -> (-13.0294, -89.1529)
  line L109 (-13.0294, -89.1529) -> (-13.5904, -89.9542)
  line L110 (-13.5904, -89.9542) -> (-13.0528, -90.7086)
  line L111 (-13.0528, -90.7086) -> (-13.5552, -90.7086)
  line L112 (-13.5552, -90.7086) -> (-13.8306, -90.2809)
  line L113 (-13.8306, -90.2809) -> (-14.1207, -90.7086)
  line L114 (-14.1207, -90.7086) -> (-14.6041, -90.7086)
  line L115 (-14.6041, -90.7086) -> (-14.0767, -89.9718)
  line L116 (-14.0767, -89.9718) -> (-14.6524, -89.1529)
  line L117 (-14.6524, -89.1529) -> (-14.147, -89.1529)
  line L118 (-14.147, -89.1529) -> (-13.8306, -89.6349)
  spline S48 degree 3 poles (-18.1431, -90.2164) (-18.1451, -90.3944) (-18.1486, -90.7033) (-18.2929, -90.9745) (-18.3541, -91.0894) knots 0 0 0 0 0.052414 0.090966 0.090966 0.090966 0.090966
  spline S49 degree 3 poles (-18.3541, -91.0894) (-18.4194, -91.1535) (-18.5544, -91.2858) (-18.7431, -91.3012) (-18.8404, -91.3092) knots 0 0 0 0 0.026595 0.054892 0.054892 0.054892 0.054892
  spline S50 degree 3 poles (-18.8404, -91.3092) (-18.9379, -91.301) (-19.1275, -91.285) (-19.2625, -91.1514) (-19.3282, -91.0865) knots 0 0 0 0 0.028347 0.055165 0.055165 0.055165 0.055165
  spline S51 degree 3 poles (-19.3282, -91.0865) (-19.3889, -90.9719) (-19.5329, -90.7002) (-19.5359, -90.3909) (-19.5377, -90.212) knots 0 0 0 0 0.038407 0.091072 0.091072 0.091072 0.091072
  spline S52 degree 3 poles (-19.5377, -90.212) (-19.5357, -90.0333) (-19.5324, -89.7234) (-19.3879, -89.4512) (-19.3267, -89.336) knots 0 0 0 0 0.052633 0.091252 0.091252 0.091252 0.091252
  spline S53 degree 3 poles (-18.335, -89.3565) (-18.2795, -89.4666) (-18.144, -89.7351) (-18.1434, -90.0377) (-18.1431, -90.2164) knots 0 0 0 0 0.036536 0.08916 0.08916 0.08916 0.08916
  spline S54 degree 3 poles (-16.4747, -90.2164) (-16.4767, -90.3944) (-16.4801, -90.7033) (-16.6244, -90.9745) (-16.6856, -91.0894) knots 0 0 0 0 0.052414 0.090966 0.090966 0.090966 0.090966
  spline S55 degree 3 poles (-16.6856, -91.0894) (-16.751, -91.1535) (-16.8859, -91.2858) (-17.0746, -91.3012) (-17.1719, -91.3092) knots 0 0 0 0 0.026595 0.054892 0.054892 0.054892 0.054892
  spline S56 degree 3 poles (-17.1719, -91.3092) (-17.2694, -91.301) (-17.4591, -91.285) (-17.5941, -91.1514) (-17.6597, -91.0865) knots 0 0 0 0 0.028347 0.055165 0.055165 0.055165 0.055165
  spline S57 degree 3 poles (-17.6597, -91.0865) (-17.7205, -90.9719) (-17.8645, -90.7002) (-17.8675, -90.3909) (-17.8692, -90.212) knots 0 0 0 0 0.038407 0.091072 0.091072 0.091072 0.091072
  spline S58 degree 3 poles (-17.8692, -90.212) (-17.8673, -90.0333) (-17.864, -89.7234) (-17.7194, -89.4512) (-17.6583, -89.336) knots 0 0 0 0 0.052633 0.091252 0.091252 0.091252 0.091252
  spline S59 degree 3 poles (-17.6583, -89.336) (-17.5929, -89.272) (-17.458, -89.1397) (-17.2692, -89.1243) (-17.1719, -89.1163) knots 0 0 0 0 0.026595 0.054892 0.054892 0.054892 0.054892
  spline S60 degree 3 poles (-17.1719, -89.1163) (-17.0727, -89.1261) (-16.8753, -89.1455) (-16.7359, -89.2865) (-16.6666, -89.3565) knots 0 0 0 0 0.028938 0.057552 0.057552 0.057552 0.057552
  spline S61 degree 3 poles (-16.6666, -89.3565) (-16.611, -89.4666) (-16.4755, -89.7351) (-16.475, -90.0377) (-16.4747, -90.2164) knots 0 0 0 0 0.036536 0.08916 0.08916 0.08916 0.08916
  line L119 (-15.5269, -91.3092) -> (-15.8609, -91.3092)
  line L120 (-15.8609, -91.3092) -> (-15.8609, -89.1529)
  line L121 (-15.8609, -89.1529) -> (-15.4493, -89.1529)
  line L122 (-15.4493, -89.1529) -> (-15.4493, -90.7042)
  spline S62 degree 3 poles (-15.4493, -90.7042) (-15.3702, -90.6383) (-15.2102, -90.505) (-15.0158, -90.43) (-14.9175, -90.3922) knots 0 0 0 0 0.030667 0.062023 0.062023 0.062023 0.062023
  line L123 (-14.9175, -90.3922) -> (-14.9175, -90.7657)
  spline S63 degree 3 poles (-14.9175, -90.7657) (-14.9747, -90.789) (-15.1, -90.8401) (-15.2086, -90.921) (-15.2676, -90.9649) knots 0 0 0 0 0.018454 0.040424 0.040424 0.040424 0.040424
  spline S64 degree 3 poles (-15.2676, -90.9649) (-15.3252, -91.015) (-15.4362, -91.1114) (-15.4974, -91.2449) (-15.5269, -91.3092) knots 0 0 0 0 0.022581 0.043539 0.043539 0.043539 0.043539
  line L124 (-30.1718, -89.1163) -> (-30.1718, -91.2638)
  line L125 (-30.1718, -91.2638) -> (-30.5937, -91.2638)
  line L126 (-30.5937, -91.2638) -> (-31.4726, -89.8297)
  line L127 (-31.4726, -89.8297) -> (-31.4726, -91.2638)
  line L128 (-31.4726, -91.2638) -> (-31.8754, -91.2638)
  line L129 (-31.8754, -91.2638) -> (-31.8754, -89.1163)
  line L130 (-25.4184, -90.9005) -> (-25.4184, -89.1163)
  line L131 (-24.9848, -89.1163) -> (-24.9848, -90.9005)
  line L132 (-24.9848, -90.9005) -> (-24.3476, -90.9005)
  line L133 (-24.3476, -90.9005) -> (-24.3476, -91.2638)
  line L134 (-24.3476, -91.2638) -> (-26.0541, -91.2638)
  line L135 (-26.0541, -91.2638) -> (-26.0541, -90.9005)
  line L136 (-26.0541, -90.9005) -> (-25.4184, -90.9005)
  line L137 (-38.9935, -91.2726) -> (-39.3275, -91.2726)
  line L138 (-39.3275, -91.2726) -> (-39.3275, -89.1163)
  line L139 (-39.3275, -89.1163) -> (-38.9159, -89.1163)
  line L140 (-38.9159, -89.1163) -> (-38.9159, -90.6676)
  spline S65 degree 3 poles (-38.9159, -90.6676) (-38.8368, -90.6017) (-38.6768, -90.4683) (-38.4824, -90.3934) (-38.3841, -90.3556) knots 0 0 0 0 0.030667 0.062023 0.062023 0.062023 0.062023
  line L141 (-38.3841, -90.3556) -> (-38.3841, -90.7291)
  spline S66 degree 3 poles (-38.3841, -90.7291) (-38.4413, -90.7524) (-38.5666, -90.8035) (-38.6752, -90.8844) (-38.7342, -90.9283) knots 0 0 0 0 0.018454 0.040424 0.040424 0.040424 0.040424
  spline S67 degree 3 poles (-38.7342, -90.9283) (-38.7918, -90.9783) (-38.9028, -91.0748) (-38.964, -91.2083) (-38.9935, -91.2726) knots 0 0 0 0 0.022581 0.043539 0.043539 0.043539 0.043539
  line L142 (-89.149, -23.75) -> (-103.049, -23.75)
  line L143 (-103.049, -23.75) -> (-103.049, -15.25)
  line L144 (-103.049, -15.25) -> (-89.149, -15.25)
  line L145 (-89.149, -15.25) -> (-89.149, -23.75)
  line L146 (-127.593, -15.208) -> (-111.193, -15.208)
  line L147 (-111.193, -15.208) -> (-111.193, -24.958)
  line L148 (-111.193, -24.958) -> (-127.593, -24.958)
  line L149 (-127.593, -24.958) -> (-127.593, -15.208)
  line L150 (-56.1296, -72.7583) -> (-39.7296, -72.7583)
  line L151 (-39.7296, -72.7583) -> (-39.7296, -82.5083)
  line L152 (-39.7296, -82.5083) -> (-56.1296, -82.5083)
  line L153 (-56.1296, -82.5083) -> (-56.1296, -72.7583)
  line L154 (-42.2616, -57.3513) -> (-42.2616, -65.8513)
  line L155 (-42.2616, -65.8513) -> (-56.1616, -65.8513)
  line L156 (-56.1616, -65.8513) -> (-56.1616, -57.3513)
  line L157 (-56.1616, -57.3513) -> (-42.2616, -57.3513)
  line L158 (-36.0196, -88.0963) -> (-36.0196, -73.5813)
  line L159 (-36.0196, -73.5813) -> (-18.8196, -73.5813)
  line L160 (-18.8196, -73.5813) -> (-18.8196, -88.0963)
  line L161 (-18.8196, -88.0963) -> (-36.0196, -88.0963)
  line L162 (-24.2714, -89.1163) -> (-23.7997, -89.1163)
  line L163 (-23.7997, -89.1163) -> (-23.6122, -89.6041)
  line L164 (-23.6122, -89.6041) -> (-22.7538, -89.6041)
  line L165 (-22.7538, -89.6041) -> (-22.5766, -89.1163)
  line L166 (-22.5766, -89.1163) -> (-22.1166, -89.1163)
  line L167 (-27.2509, -89.1163) -> (-26.8173, -89.1163)
  line L168 (-29.7997, -89.4781) -> (-29.7997, -89.1163)
  line L169 (-29.7997, -89.1163) -> (-28.1664, -89.1163)
  line L170 (-28.6, -89.4781) -> (-29.7997, -89.4781)
  spline S68 degree 3 poles (-19.3267, -89.336) (-19.2614, -89.272) (-19.1264, -89.1397) (-18.9377, -89.1243) (-18.8404, -89.1163) knots 0 0 0 0 0.026595 0.054892 0.054892 0.054892 0.054892
  spline S69 degree 3 poles (-18.8404, -89.1163) (-18.7411, -89.1261) (-18.5438, -89.1455) (-18.4043, -89.2865) (-18.335, -89.3565) knots 0 0 0 0 0.028938 0.057552 0.057552 0.057552 0.057552
  line L171 (-30.5746, -90.5167) -> (-30.5746, -89.1163)
  line L172 (-30.5746, -89.1163) -> (-30.1718, -89.1163)
  line L173 (-31.8754, -89.1163) -> (-31.4403, -89.1163)
  line L174 (-31.4403, -89.1163) -> (-30.5746, -90.5167)
  line L175 (-32.7426, -89.5279) -> (-32.7426, -89.1163)
  line L176 (-32.7426, -89.1163) -> (-32.331, -89.1163)
  line L177 (-32.331, -89.1163) -> (-32.331, -89.5279)
  line L178 (-32.331, -89.5279) -> (-32.7426, -89.5279)
  line L179 (-25.4184, -89.1163) -> (-24.9848, -89.1163)
  line L180 (-112.2444, -62.2445) -> (-112.7029, -62.2445)
  line L181 (-112.7029, -62.2445) -> (-113.5628, -60.097)
  line L182 (-113.5628, -60.097) -> (-113.0911, -60.097)
  line L183 (-113.0911, -60.097) -> (-112.9036, -60.5848)
  line L184 (-112.9036, -60.5848) -> (-112.0452, -60.5848)
  line L185 (-112.0452, -60.5848) -> (-111.868, -60.097)
  line L186 (-111.868, -60.097) -> (-111.408, -60.097)
  line L187 (-111.408, -60.097) -> (-112.2444, -62.2445)
  line L188 (-114.7098, -61.8812) -> (-114.7098, -60.097)
  line L189 (-114.7098, -60.097) -> (-114.2762, -60.097)
  line L190 (-114.2762, -60.097) -> (-114.2762, -61.8812)
  line L191 (-114.2762, -61.8812) -> (-113.639, -61.8812)
  line L192 (-113.639, -61.8812) -> (-113.639, -62.2445)
  line L193 (-113.639, -62.2445) -> (-115.3455, -62.2445)
  line L194 (-115.3455, -62.2445) -> (-115.3455, -61.8812)
  line L195 (-115.3455, -61.8812) -> (-114.7098, -61.8812)
  line L196 (-116.0603, -60.9935) -> (-116.0603, -60.097)
  line L197 (-116.0603, -60.097) -> (-115.6268, -60.097)
  line L198 (-115.6268, -60.097) -> (-115.6268, -62.2445)
  line L199 (-115.6268, -62.2445) -> (-116.5393, -62.2445)
  spline S70 degree 3 poles (-116.5393, -62.2445) (-116.639, -62.2443) (-116.808, -62.2441) (-116.9717, -62.2028) (-117.0389, -62.1859) knots 0 0 0 0 0.029736 0.050459 0.050459 0.050459 0.050459